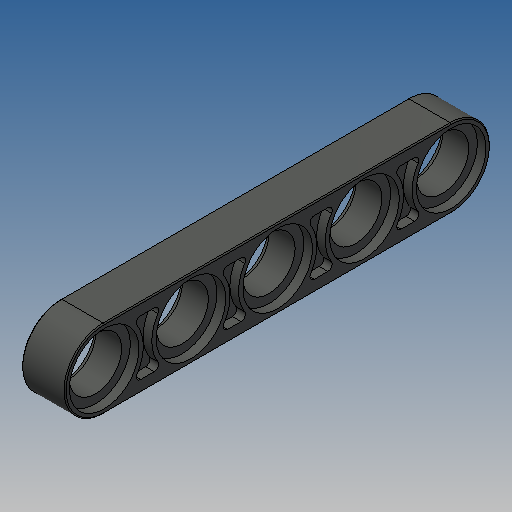
# Autodesk Inventor part: 32017-DKBluishGray
Saved by Autodesk Inventor 2025 (Build 290162010, 162A)
## iProperties
Created: 2012-03-28
Part Number: 32017-DKBluishGray
Document SubType Name: Modeling
Designer: D. Kohfeld
Density: 1.06 g/cm^3
Material: ABS Plastic
Mass: 0.616468 g
Surface Area: 11.2712 cm^2
Volume: 0.581573 cm^3
Appearance: DkBluishGray
Author: D. Kohfeld
Autodesk Inventor part; units mm, degrees
ref_plane "YZ Plane" through (0, 0, 0) normal (1, 0, 0) x (0, 1, 0)
ref_plane "XZ Plane" through (0, 0, 0) normal (0, 1, 0) x (-1, 0, 0)
ref_plane "XY Plane" through (0, 0, 0) normal (0, 0, 1) x (1, 0, 0)
sketch "Sketch3" plane through (0, 0, 0) normal (1, 0, 0) x (0, 1, 0)
  arc A0 (16, -3.6) -> (16, 3.6) centre (16, 0) ccw
  line L0 (-16, -3.6) -> (16, -3.6)
  line L1 (-16, 3.6) -> (16, 3.6)
  arc A1 (-16, 3.6) -> (-16, -3.6) centre (-16, 0) ccw
  line L2 (0, -3.6) -> (0, 3.6) construction
  circle A2 centre (-8, 0) radius 3.2
  circle A3 centre (0, 0) radius 3.2
  line L3 (0, 0) -> (-8, 0) construction
  line L4 (-8, 0) -> (-16, 0) construction
  circle A4 centre (-8, 0) radius 2.4
  circle A5 centre (0, 0) radius 2.4
  circle A6 centre (-16, 0) radius 3.2
  circle A7 centre (-16, 0) radius 2.4
  circle A8 centre (8, 0) radius 3.2
  circle A9 centre (8, 0) radius 2.4
  circle A10 centre (16, 0) radius 3.2
  circle A11 centre (16, 0) radius 2.4
  line L5 (0, 0) -> (8, 0) construction
  line L6 (8, 0) -> (16, 0) construction
  dimension "d49" = 7.2
  dimension "d59" = 6.4
  dimension "d60" = 4.8
  dimension "d64" = 8
  constraints: 14 end point, 12 centre point, 8 equal radius, 7 coincident, 4 point on circle, 4 tangent, 3 collinear, 3 equal length, 3 horizontal, 2 midpoint, 1 horizontal alignment, 1 point on line, 1 symmetric about line, 1 vertical alignment
  measures "d49" diameter of A0
  measures "d59" diameter of A2
  measures "d60" diameter of A4
  measures "d64" distance of L5.start L5.end
extrude "Extrusion4" add sketch "Sketch3" along normal mid plane 4 contours L0 A1 L1 A0 | A2 | A3 | A6 | A8 | A10
sketch "Sketch11" plane through (2, 0, 0) normal (1, 0, 0) x (0, 0, -1)
  circle A0 centre (0, 0) radius 2.4 projected
  circle A1 centre (0, -8) radius 2.4 projected
  circle A2 centre (0, 0) radius 3.2
  circle A3 centre (0, -8) radius 3.2
  circle A4 centre (0, 8) radius 2.4 projected
  arc A5 (3.6, 16) -> (-3.6, 16) centre (0, 16) ccw projected
  arc A6 (-3.6, -16) -> (3.6, -16) centre (0, -16) ccw projected
  circle A7 centre (0, -16) radius 3.2
  circle A8 centre (0, 8) radius 3.2
  circle A9 centre (0, 16) radius 3.2
  circle A10 centre (0, 16) radius 2.4 projected
  line L0 (3.6, 16) -> (3.6, -16) projected
  line L1 (-3.6, -16) -> (-3.6, 16) projected
  line L2 (-2.5456, 13.4544) -> (-2.5456, 10.5456)
  line L3 (2.5456, 13.4544) -> (2.5456, 10.5456)
  arc A11 (-2.5456, 13.4544) -> (2.5456, 13.4544) centre (0, 16) ccw
  arc A12 (2.5456, 10.5456) -> (-2.5456, 10.5456) centre (0, 8) ccw
  line L4 (0, 16) -> (-2.5456, 13.4544) construction
  line L5 (-2.5456, 5.4544) -> (-2.5456, 2.5456)
  line L6 (2.5456, 5.4544) -> (2.5456, 2.5456)
  arc A13 (-2.5456, 5.4544) -> (2.5456, 5.4544) centre (0, 8) ccw
  arc A14 (2.5456, 2.5456) -> (-2.5456, 2.5456) centre (0, 0) ccw
  line L7 (-2.5456, -2.5456) -> (-2.5456, -5.4544)
  line L8 (2.5456, -2.5456) -> (2.5456, -5.4544)
  arc A15 (-2.5456, -2.5456) -> (2.5456, -2.5456) centre (0, 0) ccw
  arc A16 (2.5456, -5.4544) -> (-2.5456, -5.4544) centre (0, -8) ccw
  line L9 (-2.5456, -10.5456) -> (-2.5456, -13.4544)
  line L10 (2.5456, -10.5456) -> (2.5456, -13.4544)
  arc A17 (-2.5456, -10.5456) -> (2.5456, -10.5456) centre (0, -8) ccw
  arc A18 (2.5456, -13.4544) -> (-2.5456, -13.4544) centre (0, -16) ccw
  dimension "d61" = 6.4
  dimension "d65" = 45
  dimension "d68" = 8
  constraints: 18 end point, 16 point on circle, 13 centre point, 7 coincident, 6 equal radius, 2 parallel, 1 horizontal alignment, 1 vertical, 30 other
  measures "d61" diameter of A3
  measures "d65" angle of L4 L1
  measures "d68" distance of L3.start L6.start
extrude "Extrusion16" cut sketch "Sketch11" against normal blind 0.8 contours A0 | A1 | A2 | A3 | A4 | A7 | A8 | A9 | A10
extrude "Extrusion17" cut sketch "Sketch11" against normal blind 0.8 contours A11 L3 A12 L2 | A13 L6 A14 L5 | A15 L8 A16 L7 | A17 L10 A18 L9
mirror "Mirror3" about plane through (0, 0, 0) normal (1, 0, 0) of "Extrusion16", "Extrusion17"
fillet "Fillet1" radius 0.1 6 edges at (-2, 19.6, 0) (-2, 0, 3.6) (-2, 0, -3.6) (2, 0, 3.6) (2, 0, -3.6) (2, 19.6, 0)
fillet "Fillet1" radius 0.4 32 edges at (1.6, -13.4544, -2.5456) (1.6, -10.5456, -2.5456) (1.6, -10.5456, 2.5456) (1.6, -13.4544, 2.5456) (1.6, -5.4544, 2.5456) (1.6, -2.5456, 2.5456) (1.6, -2.5456, -2.5456) (1.6, -5.4544, -2.5456) (1.6, 2.5456, 2.5456) (1.6, 5.4544, 2.5456) (1.6, 5.4544, -2.5456) (1.6, 2.5456, -2.5456) (1.6, 10.5456, 2.5456) (1.6, 13.4544, 2.5456) (1.6, 13.4544, -2.5456) (1.6, 10.5456, -2.5456) (-1.6, -10.5456, -2.5456) (-1.6, -13.4544, -2.5456) (-1.6, -10.5456, 2.5456) (-1.6, -13.4544, 2.5456) (-1.6, -2.5456, 2.5456) (-1.6, -5.4544, 2.5456) (-1.6, -5.4544, -2.5456) (-1.6, -2.5456, -2.5456) (-1.6, 2.5456, -2.5456) (-1.6, 5.4544, -2.5456) (-1.6, 5.4544, 2.5456) (-1.6, 2.5456, 2.5456) (-1.6, 13.4544, 2.5456) (-1.6, 10.5456, 2.5456) (-1.6, 13.4544, -2.5456) (-1.6, 10.5456, -2.5456)
equation "\"d49\" = tlad"
equation "\"d59\" = tsd"
equation "\"d60\" = tpd"
equation "\"d64\" = lu"
equation "\"d15\" = 0.5 * lu"
equation "\"d61\" = tsd"
equation "\"d68\" = lu"
equation "\"d62\" = tsl"
equation "\"d73\" = 0.5 * lu - 2 * wall"
equation "\"d56\" = lf"
equation "\"d75\" = tf"
equation "\"tlad\" = 7.2"
equation "\"tsd\" = 6.4"
equation "\"tpd\" = 4.8"
equation "\"lu\" = 8"
equation "\"tsl\" = 0.8"
equation "\"wall\" = 1.6"
equation "\"lf\" = 0.1"
equation "\"tf\" = 0.4"
body "Solid1"
